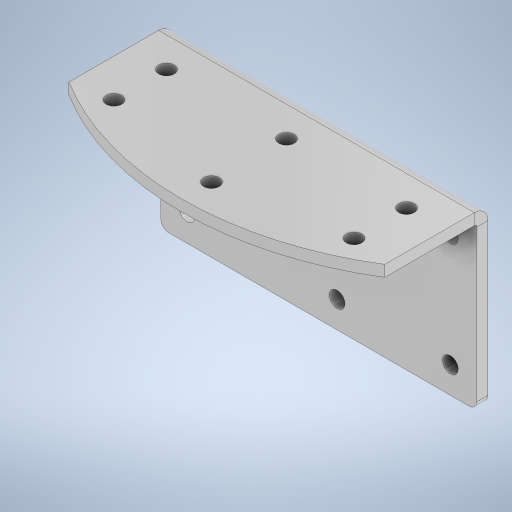
# Autodesk Inventor part: axis_2_bottom_L_frame(bottom)
Saved by Autodesk Inventor 2024.1 (Build 281209000, 209)
## iProperties
Created: 2023-09-15
Part Number: axis_2_bottom_L_frame(bottom)
Material: Aluminum 6061-AHC
Document SubType Name: Sheet Metal
Designer: chanh
Density: 2.7 g/cm^3
Sheet Metal Rule: Default_mm
Appearance: Aluminum - Dark
Author: chanh
Autodesk Inventor part; units mm, degrees
ref_plane "YZ Plane" through (0, 0, 0) normal (1, 0, 0) x (0, 1, 0)
ref_plane "XZ Plane" through (0, 0, 0) normal (0, 1, 0) x (-1, 0, 0)
ref_plane "XY Plane" through (0, 0, 0) normal (0, 0, 1) x (1, 0, 0)
sketch "Sketch1" plane through (0, 0, 0) normal (0, 0, 1) x (1, 0, 0)
  line L0 (-21.05, -11.5) -> (21.05, -11.5)
  line L1 (21.05, -11.5) -> (21.05, 11.5)
  line L2 (21.05, 11.5) -> (-21.05, 11.5)
  line L3 (-21.05, 11.5) -> (-21.05, -11.5)
  line L4 (-21.05, -11.5) -> (21.05, 11.5) construction
  line L5 (21.05, -11.5) -> (-21.05, 11.5) construction
  point P0 (0, 0)
  dimension "d0" = 42.1
  dimension "d1" = 23
  measures "d0" distance of L2.end L1.end
  measures "d1" distance of L1.end L0.end
extrude "Plate1" add sketch "Sketch1" along normal blind 1.5
sketch "Sketch2" plane through (0, 0, 1.5) normal (0, 0, 1) x (1, 0, 0)
  circle A0 centre (17.55, 7.095) radius 0.7835 projected
  circle A1 centre (17.55, -7.955) radius 0.7835 projected
  circle A2 centre (2.45, 7.095) radius 0.7835 projected
  circle A3 centre (2.45, -7.955) radius 0.7835 projected
  circle A4 centre (-17.55, 7.095) radius 0.7835 projected
  circle A5 centre (-17.55, -7.955) radius 0.7835 projected
  point P0 (0, 0)
hole "Hole1" at (17.55, -7.955, 1.5) at (2.45, -7.955, 1.5) at (-17.55, -7.955, 1.5) at (-17.55, 7.095, 1.5) at (2.45, 7.095, 1.5) at (17.55, 7.095, 1.5) direction (0, 0, -1) diameter 2.1 end through all
sketch "Sketch3" plane through (0, 0, 1.5) normal (0, 0, 1) x (1, 0, 0)
  circle A0 centre (-10.05, -0.43) radius 6.4 projected
  circle A1 centre (-10.05, -0.43) radius 6.6
  point P0 (0, 0)
  dimension "d10" = 0.2
  constraints: 1 centre point
  measures "d10" radial gap between concentric circles of A0 A1
extrude "Extrusion1" cut sketch "Sketch3" against normal through all contours A0 | A1
sketch "Sketch4" plane through (-21.05, 10, 0) normal (0, 1, 0) x (-1, 0, 0)
  line L0 (-42.1, 0) -> (0, 0)
  line L1 (0, 0) -> (0, 25)
  line L2 (0, 25) -> (-42.1, 25)
  line L3 (-42.1, 25) -> (-42.1, 0)
  constraints: 6 end point, 1 horizontal, 1 perpendicular, 1 vertical
edge flange "Flange1" height 25 angle 90 thickness 1.5 bend radius 0.31 thickness toward (0, 1, 0) relief straight relief width 1.5 relief depth 0.75 edges at (0, 11.5, 1.5) wall of the first edge with corners at (21.05, 10, 0) (-21.05, 10, 0) (-21.05, 10, 25) (21.05, 10, 25)
bend "Bend1"
corner "Corner1"
sketch "Sketch5" plane through (-21.05, 10, 25) normal (0, -1, 0) x (1, 0, 0)
  circle A0 centre (21.05, -45.25) radius 40 projected
  circle A1 centre (21.05, -45.25) radius 53
  point P0 (21.05, -25)
  dimension "d23" = 13
  constraints: 1 centre point
  measures "d23" radial gap between concentric circles of A0 A1
extrude "Cut1" cut sketch "Sketch5" against normal blind 1.5
fillet "Corner Round1" radius 1 2 edges at (21.05, -11.5, 0.75) (-21.05, -11.5, 0.75)
sketch "Sketch6" plane through (-21.05, 10, 1.81) normal (0, -1, 0) x (1, 0, 0)
  line L0 (0, 0) -> (42.1, 0) projected
  arc A0 (42.1, 11.9532) -> (0, 11.9532) centre (21.05, -22.06) ccw projected
  line L1 (21.05, 0) -> (21.05, 17.94) construction
  point P0 (21.05, -1.81)
  point P1 (5.05, 4)
  point P2 (5.05, 11)
  point P3 (21.05, 14)
  point P4 (21.05, 4)
  point P5 (37.05, 4)
  point P6 (37.05, 11)
  dimension "d27" = 10
  dimension "d28" = 4
  dimension "d29" = 16
  dimension "d30" = 7
  constraints: 3 horizontal alignment, 3 vertical alignment, 2 end point, 1 midpoint, 1 point on circle, 1 point on line, 1 symmetric about line
  measures "d27" distance of point (21.05, 14) point (21.05, 4)
  measures "d28" distance from line of point (21.05, 4) L0
  measures "d29" distance of point (37.05, 4) point (21.05, 4)
  measures "d30" distance of point (37.05, 4) point (37.05, 11)
hole "Hole2" at (-16, 10, 5.81) at (-16, 10, 12.81) at (0, 10, 15.81) at (0, 10, 5.81) at (16, 10, 5.81) at (16, 10, 12.81) direction (0, 1, 0) diameter 2.1 end through all
equation "\"d8\" = Thickness"
equation "\"d24\" = Thickness"
equation "\"d2\" = Thickness"
equation "\"d13\" = BendReliefWidth"
equation "\"d14\" = BendReliefDepth"
equation "\"d15\" = MinimumRemnant"
equation "\"d16\" = TransitionRadius"
equation "\"d19\" = BendRadius"
equation "\"d20\" = CornerReliefSize"
equation "\"d21\" = GapSize"
equation "\"d22\" = JacobiRadiusSize"
equation "\"BendReliefWidth\" = Thickness"
equation "\"BendReliefDepth\" = 0.5 * Thickness"
equation "\"CornerReliefSize\" = 4 * Thickness"
equation "\"MinimumRemnant\" = 2 * Thickness"
equation "\"TransitionRadius\" = BendRadius"
equation "\"JacobiRadiusSize\" = BendRadius"
equation "\"GapSize\" = Thickness"
equation "\"Thickness\" = 1.5"
equation "\"BendRadius\" = 0.31"
body "Solid1"
